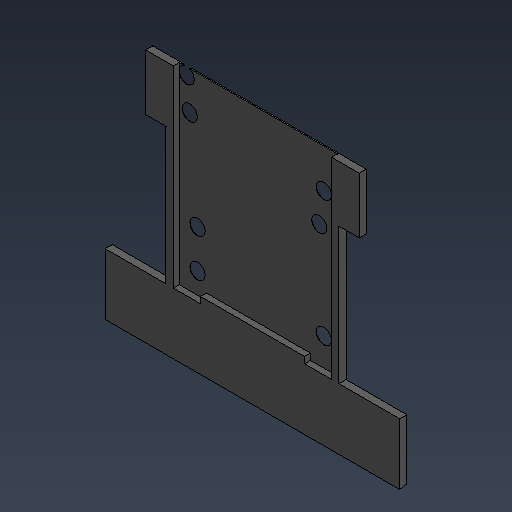
# Autodesk Inventor part: Ceiling
Saved by Autodesk Inventor 2026.2 (Build 302298010, 298A)
## iProperties
Created: 2026-04-07
Part Number: Ceiling
Material: Generic
Document SubType Name: Modeling
Designer: szymo
Density: 1 g/cm^3
Appearance: Default(1)
Author: szymo
Autodesk Inventor part; units mm, degrees
ref_plane "YZ Plane" through (0, 0, 0) normal (1, 0, 0) x (0, 1, 0)
ref_plane "XZ Plane" through (0, 0, 0) normal (0, 1, 0) x (-1, 0, 0)
ref_plane "XY Plane" through (0, 0, 0) normal (0, 0, 1) x (1, 0, 0)
sketch "Sketch1" plane through (0, 0, 0) normal (0, 0, 1) x (1, 0, 0)
  line L0 (-14.25, -14.5) -> (13.65, -14.5)
  line L1 (-13.65, -55.2958) -> (14.25, -55.2958)
  line L2 (50, 0) -> (-50, 0)
  line L3 (-50, 0) -> (-50, -90)
  line L4 (-50, -90) -> (50, -90)
  line L5 (50, -90) -> (50, 0)
  line L6 (50, -86.2958) -> (-50, -86.2958)
  line L7 (14.65, -6.65) -> (-15.25, -6.65)
  line L8 (-15.25, -6.65) -> (-15.25, -22.35)
  line L9 (-15.25, -22.35) -> (14.65, -22.35)
  line L10 (14.65, -22.35) -> (14.65, -6.65)
  line L11 (15.25, -47.4458) -> (-14.65, -47.4458)
  line L12 (-14.65, -47.4458) -> (-14.65, -63.1458)
  line L13 (-14.65, -63.1458) -> (15.25, -63.1458)
  line L14 (15.25, -63.1458) -> (15.25, -47.4458)
  line L15 (30.5, -65.2958) -> (29.35, -65.2958)
  line L16 (-30.5, -65.2958) -> (-29.35, -65.2958)
  circle A0 centre (20.65, -24.0677) radius 2.25 projected
  circle A1 centre (22.6692, -56.1259) radius 2.25 projected
  circle A2 centre (22.25, -13.4966) radius 2.25 projected
  line L17 (19.75, -61.0677) -> (19.75, -50.9236) projected
  line L18 (19.75, -50.9236) -> (23.15, -50.9236) projected
  line L19 (23.15, -50.9236) -> (23.15, -46.7261) projected
  line L20 (19.75, -46.7261) -> (23.15, -46.7261) projected
  line L21 (19.75, -46.7261) -> (19.75, -44.8549) projected
  line L22 (19.75, -44.8549) -> (17.65, -44.8549) projected
  line L23 (17.65, 0) -> (17.65, -44.8549) projected
  line L24 (17.65, 0) -> (26.85, 0) projected
  line L25 (26.85, -65.2958) -> (26.85, 0) projected
  line L26 (23.15, -65.2958) -> (26.85, -65.2958) projected
  line L27 (23.15, -65.2958) -> (23.15, -61.0677) projected
  line L28 (19.75, -61.0677) -> (23.15, -61.0677) projected
  circle A3 centre (-24.3428, -2.5072) radius 2.25 projected
  circle A4 centre (-20.65, -57.8419) radius 2.25 projected
  circle A5 centre (-20.65, -44.9257) radius 2.25 projected
  circle A6 centre (-23.3, -12.9282) radius 2.25 projected
  line L29 (-26.85, 0) -> (-17.65, 0) projected
  line L30 (-17.65, -4.0591) -> (-17.65, 0) projected
  line L31 (-19.75, -4.0591) -> (-17.65, -4.0591) projected
  line L32 (-19.75, -4.7124) -> (-19.75, -4.0591) projected
  line L33 (-19.75, -4.7124) -> (-23.15, -4.7124) projected
  line L34 (-23.15, -4.7124) -> (-23.15, -8.7282) projected
  line L35 (-19.75, -8.7282) -> (-23.15, -8.7282) projected
  line L36 (-19.75, -18.8723) -> (-19.75, -8.7282) projected
  line L37 (-19.75, -18.8723) -> (-23.15, -18.8723) projected
  line L38 (-23.15, -18.8723) -> (-23.15, -23.0697) projected
  line L39 (-19.75, -23.0697) -> (-23.15, -23.0697) projected
  line L40 (-19.75, -24.9409) -> (-19.75, -23.0697) projected
  line L41 (-19.75, -24.9409) -> (-17.65, -24.9409) projected
  line L42 (-17.65, -65.2958) -> (-17.65, -24.9409) projected
  line L43 (-26.85, -65.2958) -> (-17.65, -65.2958) projected
  line L44 (-26.85, 0) -> (-26.85, -65.2958) projected
  line L45 (-17.65, -4.0591) -> (-17.65, -24.9409)
  line L46 (23.15, -65.2958) -> (17.65, -65.2958)
  line L47 (17.65, -65.2958) -> (17.65, -44.8549)
  line L48 (17.65, -6.65) -> (-17.65, -6.65)
  line L49 (-17.65, -63.1458) -> (17.65, -63.1458)
  line L50 (-26.85, -65.2958) -> (-26.85, -13) projected
  line L51 (-26.85, -65.2958) -> (-29.35, -65.2958) projected
  line L52 (-29.35, -65.2958) -> (-29.35, -19) projected
  line L53 (-29.35, -19) -> (-36.25, -19) projected
  line L54 (-36.25, -13) -> (-36.25, -19) projected
  line L55 (-26.85, -13) -> (-36.25, -13) projected
  line L56 (26.85, -13) -> (26.85, -65.2958) projected
  line L57 (26.85, -13) -> (36.25, -13) projected
  line L58 (36.25, -19) -> (36.25, -13) projected
  line L59 (29.35, -19) -> (36.25, -19) projected
  line L60 (29.35, -19) -> (29.35, -65.2958) projected
  line L61 (29.35, -65.2958) -> (26.85, -65.2958) projected
  line L62 (-26.85, -3) -> (-26.85, 0) projected
  line L63 (-26.85, -3) -> (-36.25, -3) projected
  line L64 (-36.25, 0) -> (-36.25, -3) projected
  line L65 (-26.85, 0) -> (-36.25, 0) projected
  line L66 (26.85, 0) -> (26.85, -3) projected
  line L67 (26.85, 0) -> (36.25, 0) projected
  line L68 (36.25, -3) -> (36.25, 0) projected
  line L69 (26.85, -3) -> (36.25, -3) projected
  arc A7 (26.85, -66.2958) -> (29.85, -69.2958) centre (29.85, -66.2958) ccw projected
  line L70 (26.85, -65.2958) -> (26.85, -66.2958) projected
  line L71 (26.85, -65.2958) -> (50, -65.2958) projected
  line L72 (50, -65.2958) -> (50, -85.9433) projected
  line L73 (34.5, -85.9433) -> (50, -85.9433) projected
  line L74 (34.5, -78.442) -> (34.5, -85.9433) projected
  line L75 (34.5, -78.442) -> (45.421, -78.442) projected
  arc A8 (45.421, -78.442) -> (46.8031, -78.442) centre (46.112, -80.4779) ccw projected
  line L76 (46.8031, -78.442) -> (49, -78.442) projected
  line L77 (49, -78.442) -> (49, -69.922) projected
  line L78 (49, -69.922) -> (46.525, -69.922) projected
  line L79 (46.525, -69.922) -> (32.6782, -69.3038) projected
  arc A9 (32.6782, -69.3038) -> (32.5, -69.2958) centre (32.5, -71.2958) ccw projected
  line L80 (32.5, -69.2958) -> (29.85, -69.2958) projected
  arc A10 (-29.85, -69.2958) -> (-26.85, -66.2958) centre (-29.85, -66.2958) ccw projected
  line L81 (-32.5, -69.2958) -> (-29.85, -69.2958) projected
  arc A11 (-32.5, -69.2958) -> (-32.6782, -69.3038) centre (-32.5, -71.2958) ccw projected
  line L82 (-32.6782, -69.3038) -> (-46.525, -69.922) projected
  line L83 (-46.525, -69.922) -> (-49, -69.922) projected
  line L84 (-49, -69.922) -> (-49, -78.442) projected
  line L85 (-49, -78.442) -> (-46.8031, -78.442) projected
  arc A12 (-46.8031, -78.442) -> (-45.421, -78.442) centre (-46.112, -80.4779) ccw projected
  line L86 (-45.421, -78.442) -> (-34.5, -78.442) projected
  line L87 (-34.5, -78.442) -> (-34.5, -85.9433) projected
  line L88 (-34.5, -85.9433) -> (-50, -85.9433) projected
  line L89 (-50, -65.2958) -> (-50, -85.9433) projected
  line L90 (-26.85, -65.2958) -> (-50, -65.2958) projected
  line L91 (-26.85, -65.2958) -> (-26.85, -66.2958) projected
  line L92 (36.25, 0) -> (36.25, -19)
  line L93 (-36.25, -19) -> (-36.25, 0)
  point P0 (0, 0)
  point P1 (26.95, 0)
  point P2 (-15.25, -6.65)
  dimension "d0" = 50
  dimension "d1" = 50
  dimension "d2" = 90
  dimension "d3" = 7.85
  dimension "d4" = 7.85
  dimension "d5" = 1
  dimension "d6" = 1
  dimension "d7" = 7.85
  dimension "d8" = 7.85
  dimension "d9" = 1
  dimension "d10" = 1
  dimension "d21" = 0
  constraints: 46 end point, 8 horizontal, 5 parallel, 5 perpendicular, 5 point on line, 4 vertical, 1 collinear, 8 other
  measures "d0" distance from line of L5 point (0, 0)
  measures "d1" distance from line of L3 point (0, 0)
  measures "d2" distance of the line from the sketch origin of L4
  measures "d3" distance between parallel lines of L11 L1
  measures "d4" distance between parallel lines of L13 L1
  measures "d5" distance from line of L14 L1.end
  measures "d6" distance from line of L12 L1.start
  measures "d7" distance between parallel lines of L7 L0
  measures "d8" distance between parallel lines of L9 L0
  measures "d9" distance from line of L10 L0.end
  measures "d10" distance from line of L8 L0.start
  measures "d21" distance between parallel lines of L13 L49
extrude "Extrusion4" add sketch "Sketch1" along normal blind 2 contours L68 L69 L25 L2 | L5 L73 L74 L75 A8 L76 L77 L78 L79 A9 L80 A7 L70 L61 L15 L71 | L92 L57 L25 L69 | L5 L6 L3 L88 L87 L86 A12 L85 L84 L83 L82 A11 L81 A10 L91 L43 L42 L49 L13 L47 L46 L26 L70 A7 L80 A9 L79 L78 L77 L76 A8 L75 L74 L73 | L58 L59 L60 L61 L25 L57 | L44 L63 L64 L2 | L3 L90 L16 L51 L91 A10 L81 A11 L82 L83 L84 L85 A12 L86 L87 L88 | L44 L55 L93 L63 | L44 L51 L52 L53 L54 L55
extrude "Extrusion5" add sketch "Sketch1" against normal blind 0.4 contours L68 L69 L25 L2 | L5 L73 L74 L75 A8 L76 L77 L78 L79 A9 L80 A7 L70 L61 L15 L71 | L25 L26 L27 L28 L17 L18 L19 L20 L21 L22 L23 L2 | L92 L57 L25 L69 | L5 L6 L3 L88 L87 L86 A12 L85 L84 L83 L82 A11 L81 A10 L91 L43 L42 L49 L13 L47 L46 L26 L70 A7 L80 A9 L79 L78 L77 L76 A8 L75 L74 L73 | L23 L48 L7 L45 L30 L2 | L58 L59 L60 L61 L25 L57 | L30 L31 L32 L33 L34 L35 L36 L37 L38 L39 L40 L41 L42 L43 L44 L2 | L23 L47 L49 L14 L11 L12 L42 L45 L48 L8 L9 L10 | L44 L63 L64 L2 | L45 L41 L40 L39 L38 L37 L36 L35 L34 L33 L32 L31 | L22 L21 L20 L19 L18 L17 L28 L27 L46 L47 | L10 L9 L8 L7 | L3 L90 L16 L51 L91 A10 L81 A11 L82 L83 L84 L85 A12 L86 L87 L88 | L44 L55 L93 L63 | L44 L51 L52 L53 L54 L55 | L13 L12 L11 L14 | A0 | A1 | A2 | A3 | A4 | A5 | A6
sketch "Sketch2" plane through (50, -86.2958, 2) normal (1, 0, 0) x (0, 0, -1)
  line L0 (2.2133, 0.4205) -> (-23.8, -4.5217) projected
  line L1 (-23.8, -4.5217) -> (-23.6133, -5.5042) projected
  line L2 (-23.6133, -5.5042) -> (2.4, -0.5619) projected
  line L3 (2.4, -0.5619) -> (2.2133, 0.4205) projected
  line L4 (0, -10.5619) -> (0, 0.2036)
  line L5 (0, 0.2036) -> (2.4, 0.6596)
  line L6 (2.4, 0.6596) -> (2.4, -10.5619)
  line L7 (2.4, -10.5619) -> (0, -10.5619)
  point P0 (2, 86.2958)
  dimension "d15" = 2.4
  dimension "d16" = 0.2
  dimension "d17" = 0
  dimension "d18" = 10
  constraints: 8 end point, 2 vertical, 1 parallel, 1 perpendicular
  measures "d15" distance from line of L4 L2.end
  measures "d16" distance between parallel lines of L5 L0
  measures "d17" distance from line of L6 L2.end
  measures "d18" distance from line of L7 L2.end
extrude "Extrusion3" cut sketch "Sketch2" against normal through all contours L3 L2 L4 L0 | L0 L4 L5 L6 L3 | L6 L7 L4 L2
sketch "Sketch3" plane through (0, 0, -0.4) normal (0, 0, -1) x (-1, 0, 0)
  circle A0 centre (24.3428, -2.5072) radius 1.5 projected
  circle A1 centre (23.3, -12.9282) radius 1.5 projected
  circle A2 centre (20.65, -58.1775) radius 1.5 projected
  circle A3 centre (20.65, -45.2613) radius 1.5 projected
  circle A4 centre (-20.65, -23.7673) radius 1.5 projected
  circle A5 centre (-22.25, -55.8509) radius 1.5 projected
  circle A6 centre (-22.253, -13.1962) radius 1.5 projected
  arc A7 (-26.256, -0.1) -> (-26.756, -0.6) centre (-26.256, -0.6) ccw projected
  line L0 (-26.756, -0.6) -> (-26.756, -64.6958) projected
  arc A8 (-26.756, -64.6958) -> (-26.256, -65.1958) centre (-26.256, -64.6958) ccw projected
  line L1 (-26.256, -65.1958) -> (-23.756, -65.1958) projected
  arc A9 (-23.756, -65.1958) -> (-23.256, -64.6958) centre (-23.756, -64.6958) ccw projected
  line L2 (-23.256, -64.6958) -> (-23.256, -61.4677) projected
  arc A10 (-22.756, -60.9677) -> (-23.256, -61.4677) centre (-22.756, -61.4677) ccw projected
  line L3 (-22.756, -60.9677) -> (-20.35, -60.9677) projected
  arc A11 (-20.35, -60.9677) -> (-19.85, -60.4677) centre (-20.35, -60.4677) ccw projected
  line L4 (-19.85, -60.4677) -> (-19.85, -51.8592) projected
  arc A12 (-19.85, -51.8592) -> (-20.35, -51.3592) centre (-20.35, -51.8592) ccw projected
  line L5 (-20.35, -51.3592) -> (-22.756, -51.3592) projected
  arc A13 (-23.256, -50.8592) -> (-22.756, -51.3592) centre (-22.756, -50.8592) ccw projected
  line L6 (-23.256, -50.8592) -> (-23.256, -41.5958) projected
  arc A14 (-22.756, -41.0958) -> (-23.256, -41.5958) centre (-22.756, -41.5958) ccw projected
  line L7 (-22.756, -41.0958) -> (-12.25, -41.0958) projected
  arc A15 (-11.75, -41.5958) -> (-12.25, -41.0958) centre (-12.25, -41.5958) ccw projected
  line L8 (-11.75, -41.5958) -> (-11.75, -43.0958) projected
  arc A16 (-11.75, -43.0958) -> (-11.25, -43.5958) centre (-11.25, -43.0958) ccw projected
  line L9 (-11.25, -43.5958) -> (11.25, -43.5958) projected
  arc A17 (11.25, -43.5958) -> (11.75, -43.0958) centre (11.25, -43.0958) ccw projected
  line L10 (11.75, -43.0958) -> (11.75, -41.5958) projected
  arc A18 (12.25, -41.0958) -> (11.75, -41.5958) centre (12.25, -41.5958) ccw projected
  line L11 (12.25, -41.0958) -> (17.25, -41.0958) projected
  arc A19 (17.75, -41.5958) -> (17.25, -41.0958) centre (17.25, -41.5958) ccw projected
  line L12 (17.75, -41.5958) -> (17.75, -64.6958) projected
  arc A20 (17.75, -64.6958) -> (18.25, -65.1958) centre (18.25, -64.6958) ccw projected
  line L13 (18.25, -65.1958) -> (26.25, -65.1958) projected
  arc A21 (26.25, -65.1958) -> (26.75, -64.6958) centre (26.25, -64.6958) ccw projected
  line L14 (26.75, -64.6958) -> (26.75, -0.6) projected
  arc A22 (26.75, -0.6) -> (26.25, -0.1) centre (26.25, -0.6) ccw projected
  line L15 (26.25, -0.1) -> (18.25, -0.1) projected
  arc A23 (18.25, -0.1) -> (17.75, -0.6) centre (18.25, -0.6) ccw projected
  line L16 (17.75, -0.6) -> (17.75, -3.1235) projected
  arc A24 (17.75, -3.1235) -> (18.25, -3.6235) centre (18.25, -3.1235) ccw projected
  line L17 (18.25, -3.6235) -> (22.75, -3.6235) projected
  arc A25 (23.25, -4.1235) -> (22.75, -3.6235) centre (22.75, -4.1235) ccw projected
  line L18 (23.25, -4.1235) -> (23.25, -8.3282) projected
  arc A26 (22.75, -8.8282) -> (23.25, -8.3282) centre (22.75, -8.3282) ccw projected
  line L19 (22.75, -8.8282) -> (20.35, -8.8282) projected
  arc A27 (20.35, -8.8282) -> (19.85, -9.3282) centre (20.35, -9.3282) ccw projected
  line L20 (19.85, -9.3282) -> (19.85, -17.9366) projected
  arc A28 (19.85, -17.9366) -> (20.35, -18.4366) centre (20.35, -17.9366) ccw projected
  line L21 (20.35, -18.4366) -> (22.75, -18.4366) projected
  arc A29 (23.25, -18.9366) -> (22.75, -18.4366) centre (22.75, -18.9366) ccw projected
  line L22 (23.25, -18.9366) -> (23.25, -28.2) projected
  arc A30 (22.75, -28.7) -> (23.25, -28.2) centre (22.75, -28.2) ccw projected
  line L23 (22.75, -28.7) -> (12.25, -28.7) projected
  arc A31 (11.75, -28.2) -> (12.25, -28.7) centre (12.25, -28.2) ccw projected
  line L24 (11.75, -28.2) -> (11.75, -26.7) projected
  arc A32 (11.75, -26.7) -> (11.25, -26.2) centre (11.25, -26.7) ccw projected
  line L25 (11.25, -26.2) -> (-17.25, -26.2) projected
  arc A33 (-17.75, -25.7) -> (-17.25, -26.2) centre (-17.25, -25.7) ccw projected
  line L26 (-17.75, -25.7) -> (-17.75, -0.6) projected
  arc A34 (-17.75, -0.6) -> (-18.25, -0.1) centre (-18.25, -0.6) ccw projected
  line L27 (-18.25, -0.1) -> (-26.256, -0.1) projected
  line L28 (-29.5, -65.8371) -> (-50, -65.8371) projected
  line L29 (-50, -65.8371) -> (-50, -86.3723) projected
  line L30 (-34.5, -86.3723) -> (-50, -86.3723) projected
  line L31 (-34.5, -78.883) -> (-34.5, -86.3723) projected
  line L32 (-34.5, -78.883) -> (-49, -78.883) projected
  line L33 (-49, -70.278) -> (-33.7527, -70.278) projected
  line L34 (-32.5, -69.8371) -> (-31.5, -69.8371) projected
  line L35 (29.5, -65.8371) -> (50, -65.8371) projected
  line L36 (33.7527, -70.278) -> (49, -70.278) projected
  line L37 (49, -78.883) -> (34.5, -78.883) projected
  circle A35 centre (-47.662, -81.0191) radius 2.15 projected
  circle A36 centre (-46.75, -80.983) radius 2.05 projected
  line L38 (34.5, -78.883) -> (34.5, -86.3723) projected
  line L39 (29.5, -67.8371) -> (29.5, -65.8371) projected
  arc A37 (29.5, -67.8371) -> (31.5, -69.8371) centre (31.5, -67.8371) ccw projected
  line L40 (32.5, -69.8371) -> (31.5, -69.8371) projected
  arc A38 (33.7527, -70.278) -> (32.5, -69.8371) centre (32.5, -71.8371) ccw projected
  arc A39 (-31.5, -69.8371) -> (-29.5, -67.8371) centre (-31.5, -67.8371) ccw projected
  line L41 (-29.5, -67.8371) -> (-29.5, -65.8371) projected
  arc A40 (-32.5, -69.8371) -> (-33.7527, -70.278) centre (-32.5, -71.8371) ccw projected
  line L42 (-49, -78.883) -> (-49, -70.278) projected
  line L43 (49, -70.278) -> (49, -78.883) projected
  line L44 (34.5, -86.3723) -> (50, -86.3723) projected
  line L45 (50, -65.8371) -> (50, -86.3723) projected
  circle A41 centre (46.75, -80.983) radius 2.05 projected
  point P0 (0, 0)
  point P1 (-49, -78.442)
  point P2 (-49, -78.292)
  point P3 (-50, -86.5495)
  point P4 (-34.5, -86.5495)
  point P5 (-50, -66.2871)
  point P6 (-34.5, -78.8554)
  point P7 (-49, -70.3354)
  point P8 (49, -78.2054)
  point P9 (49, -77.792)
  point P10 (36.05, -86.3723)
hole "Hole1" at (22.25, -55.8509, -0.4) at (20.65, -23.7673, -0.4) at (22.253, -13.1962, -0.4) at (-24.3428, -2.5072, -0.4) at (-23.3, -12.9282, -0.4) at (-20.65, -45.2613, -0.4) at (-20.65, -58.1775, -0.4) direction (0, 0, 1) diameter 3.4 depth 10 countersink diameter 6 countersink angle 90 clearance for "Countersunk Flat Head Screw ISO 2009/7046" size "M3" standard "ISO"
equation "\"d4\" = d3"
equation "\"d6\" = d5"
equation "\"d7\" = d3"
equation "\"d8\" = d3"
equation "\"d9\" = d5"
equation "\"d10\" = d5"
body "Solid1"
